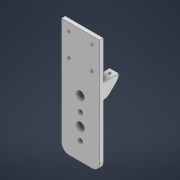
# Autodesk Inventor part: 3d mount for linear bearing
Saved by Autodesk Inventor 2021 (Build 250183000, 183)
## iProperties
Created: 2022-05-25
Part Number: 3d mount for linear bearing
Material: Generic
Document SubType Name: Modeling
Designer: techv
Density: 1 g/cm^3
Appearance: Default
Author: techv
Autodesk Inventor part; units mm, degrees
ref_plane "YZ Plane" through (0, 0, 0) normal (1, 0, 0) x (0, 1, 0)
ref_plane "XZ Plane" through (0, 0, 0) normal (0, 1, 0) x (-1, 0, 0)
ref_plane "XY Plane" through (0, 0, 0) normal (0, 0, 1) x (1, 0, 0)
sketch "Sketch1" plane through (0, 0, 0) normal (0, 0, 1) x (1, 0, 0)
  line L0 (25, 11) -> (-25, 11) projected
  line L1 (-25, 61) -> (25, 61)
  line L2 (25, 61) -> (25, -39)
  line L3 (25, -39) -> (-25, -39)
  line L4 (-25, -39) -> (-25, 61)
  line L5 (-25, 61) -> (25, -39) construction
  line L6 (25, 61) -> (-25, -39) construction
  line L7 (25, -39) -> (-25, -39)
  line L8 (-25, -39) -> (-25, -89)
  line L9 (-25, -89) -> (25, -89)
  line L10 (25, -89) -> (25, -39)
  point P0 (0, 0)
  point P1 (0, 11)
  dimension "d0" = 50
  dimension "d1" = 100
  dimension "d2" = 50
  dimension "d3" = 50
  constraints: 20 end point, 4 parallel, 3 midpoint, 2 horizontal, 2 perpendicular
  measures "d0" distance of L2.end L3.end
  measures "d1" distance of L1.end L2.end
  measures "d2" distance of L9.end L8.end
  measures "d3" distance of L8.end L7.end
extrude "Extrusion1" add sketch "Sketch1" along normal blind 5
fillet "Fillet1" radius 10 2 edges at (25, -89, 2.5) (-25, -89, 2.5)
ref_plane "Work Plane1" through (-15, 11, 0) normal (0, -1, 0) x (1, 0, 0)
sketch "Sketch2" plane through (-15, 11, 0) normal (0, -1, 0) x (1, 0, 0)
  line L0 (40, -0.5) -> (-10, -0.5) projected
  line L1 (-10, -0.5) -> (-10, -3.5) projected
  line L2 (40, -3.5) -> (-10, -3.5) projected
  line L3 (40, -0.5) -> (40, -3.5) projected
  line L4 (-10, -3.5) -> (40, -3.5) projected
  line L5 (-10, -3.5) -> (-10, -53.5) projected
  line L6 (-10, -53.5) -> (40, -53.5) projected
  line L7 (40, -53.5) -> (40, -3.5) projected
  line L8 (40, -3.5) -> (-10, -3.5) projected
  ellipse E0 centre (15, -28.5) end of major axis (18.5, -28.5) minor radius 3.5 projected
  line L9 (-10, 0) -> (0, 0) projected
  line L10 (40, 0) -> (-10, 0) projected
  line L11 (30, 0) -> (40, 0) projected
  line L12 (0, 0) -> (30, 0) projected
  line L13 (25, -0.5) -> (5, -0.5) projected
  line L14 (5, -0.5) -> (5, -20.5) projected
  line L15 (25, -20.5) -> (5, -20.5) projected
  line L16 (25, -0.5) -> (25, -20.5) projected
  line L17 (40, 0) -> (28, 0)
  line L18 (28, 0) -> (28, -20)
  line L19 (28, -20) -> (40, -20)
  line L20 (40, -20) -> (40, 0)
  line L21 (-10, 0) -> (2, 0)
  line L22 (2, 0) -> (2, -20)
  line L23 (2, -20) -> (-10, -20)
  line L24 (-10, -20) -> (-10, 0)
  point P0 (15, 0)
  dimension "d8" = 12
  dimension "d9" = 20
  dimension "d10" = 12
  dimension "d11" = 20
  constraints: 16 end point, 4 parallel, 2 horizontal, 2 perpendicular
  measures "d8" distance of L19.end L18.end
  measures "d9" distance of L18.end L17.end
  measures "d10" distance of L22.end L23.end
  measures "d11" distance of L21.end L22.end
extrude "Extrusion2" add sketch "Sketch2" along normal blind 20 contours L18 L10 L20 L0 | L0 L3 L2 L18 | L22 L2 L1 L0 | L0 L24 L9 L10 L22 | L2 L7 L19 L18 | L22 L23 L5 L2
chamfer "Chamfer1" distance 15 angle 45 2 edges at (-19, -9, -20) (19, -9, -20)
fillet "Fillet2" radius 10 2 edges at (-19, 6, -20) (-19, -9, -5)
fillet "Fillet3" radius 10 2 edges at (19, -9, -5) (19, 6, -20)
sketch "Sketch3" plane through (0, 0, 5) normal (0, 0, 1) x (1, 0, 0)
  line L0 (25, -79) -> (25, 61) projected
  line L1 (-25, 61) -> (-25, -79) projected
  line L2 (25, 61) -> (-25, 61)
  line L3 (-25, 61) -> (-25, 11)
  line L4 (-25, 11) -> (25, 11)
  line L5 (25, 11) -> (25, 61)
  line L6 (-15, 51) -> (15, 51)
  line L7 (15, 51) -> (15, 21)
  line L8 (15, 21) -> (-15, 21)
  line L9 (-15, 21) -> (-15, 51)
  line L10 (-15, 51) -> (15, 21) construction
  line L11 (15, 51) -> (-15, 21) construction
  circle A0 centre (15, 21) radius 1.5
  circle A1 centre (15, 51) radius 1.5
  circle A2 centre (-15, 51) radius 1.5
  circle A3 centre (-15, 21) radius 1.5
  point P0 (0, 0)
  point P1 (0, 36)
  dimension "d19" = 50
  dimension "d20" = 30
  dimension "d21" = 30
  dimension "d22" = 3
  dimension "d23" = 3
  dimension "d24" = 3
  dimension "d25" = 3
  constraints: 20 end point, 4 centre point, 4 coincident, 4 parallel, 2 horizontal, 2 midpoint, 2 perpendicular, 1 point on line
  measures "d19" distance of L3.end L2.end
  measures "d20" distance of L7.end L8.end
  measures "d21" distance of L6.end L7.end
  measures "d22" diameter of A0
  measures "d23" diameter of A1
  measures "d24" diameter of A2
  measures "d25" diameter of A3
extrude "Extrusion3" cut sketch "Sketch3" against normal blind 20 contours L9 A2 L6 | L6 A2 L9 | A1 L7 L6 | L6 L7 A1 | A3 L8 L9 | L9 L8 A3 | A0 L8 L7 | L7 L8 A0
sketch "Sketch4" plane through (-15, 11, 0) normal (0, 1, 0) x (1, 0, 0)
  line L0 (-10, 0) -> (-10, 20) projected
  line L1 (-10, 20) -> (2, 20)
  line L2 (2, 20) -> (2, 8)
  line L3 (2, 8) -> (-10, 8)
  line L4 (-10, 8) -> (-10, 20)
  circle A0 centre (-4, 14) radius 1.5
  circle A1 centre (34, 14) radius 1.5
  point P0 (15, 0)
  dimension "d28" = 12
  dimension "d29" = 12
  dimension "d30" = 3
  dimension "d33" = 38
  constraints: 8 end point, 2 centre point, 2 horizontal, 2 parallel, 1 perpendicular, 2 other
  measures "d28" distance of L2.end L3.end
  measures "d29" distance of L1.end L2.end
  measures "d30" diameter of A0
  measures "d33" distance of A0.centre A1.centre
extrude "Extrusion4" cut sketch "Sketch4" against normal through all contours A0 | A1
sketch "Sketch5" plane through (-15, -9, 0) normal (0, -1, 0) x (1, 0, 0)
  circle A0 centre (34, -14) radius 1.5 projected
  circle A1 centre (-4, -14) radius 1.5 projected
  circle A2 centre (34, -14) radius 2.5
  circle A3 centre (-4, -14) radius 1.5 projected
  circle A4 centre (-4, -14) radius 2.5
  point P0 (15, 0)
  dimension "d40" = 5
  dimension "d41" = 5
  constraints: 2 centre point, 2 coincident
  measures "d40" diameter of A2
  measures "d41" diameter of A4
extrude "Extrusion5" cut sketch "Sketch5" against normal blind 15
sketch "Sketch6" plane through (0, 0, 5) normal (0, 0, 1) x (1, 0, 0)
  circle A0 centre (0, -49) radius 5
  line L0 (25, 61) -> (-25, 61) projected
  circle A1 centre (0, -32.75) radius 2.6
  circle A2 centre (0, -65.25) radius 2.6
  circle A3 centre (0, -14) radius 5
  point P0 (0, 0)
  dimension "d44" = 10
  dimension "d45" = 110
  dimension "d46" = 5.2
  dimension "d47" = 5.2
  dimension "d48" = 16.25
  dimension "d49" = 16.25
  dimension "d52" = 10
  dimension "d53" = 75
  constraints: 4 centre point
  measures "d44" diameter of A0
  measures "d45" distance from line of L0 A0.centre
  measures "d46" diameter of A1
  measures "d47" diameter of A2
  measures "d48" distance of A1.centre A0.centre
  measures "d49" distance of A0.centre A2.centre
  measures "d52" diameter of A3
  measures "d53" distance from line of L0 A3.centre
extrude "Extrusion6" cut sketch "Sketch6" against normal blind 10
body "Solid1"
